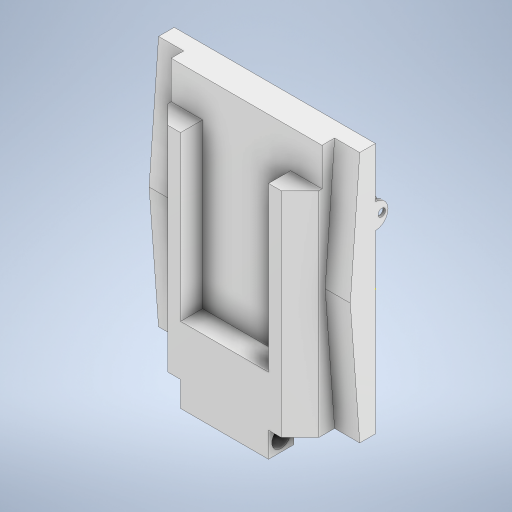
# Autodesk Inventor part: Hebeteil
Saved by Autodesk Inventor 2023 (Build 270158000, 158)
## iProperties
Created: 2024-02-03
Part Number: Hebeteil
Material: Acetalharz, Weiß
Document SubType Name: Modeling
Designer: jefar
Density: 1.425 g/cm^3
Appearance: Glatt - Weiß
Mass: 1.50722e+08 g
Surface Area: 2.46257e+06 cm^2
Volume: 1.0577e+08 cm^3
Author: jefar
Autodesk Inventor part; units mm, degrees
ref_plane "YZ Plane" through (0, 0, 0) normal (1, 0, 0) x (0, 1, 0)
sketch "Skizze1" plane through (0, 0, 0) normal (0, 0, 1) x (1, 0, 0)
  line L0 (-5600, 0) -> (5600, 0) construction
  line L1 (0, -7000) -> (0, 7000) construction
  line L2 (-4000, -5000) -> (4000, -5000)
  line L3 (4000, -5000) -> (4000, 5000)
  line L4 (4000, 5000) -> (-4000, 5000)
  line L5 (-4000, 5000) -> (-4000, -5000)
  line L6 (-4000, -5000) -> (4000, 5000) construction
  line L7 (4000, -5000) -> (-4000, 5000) construction
  point P0 (0, 0)
  dimension "d0" = 8000
  dimension "d1" = 10000
  constraints: 12 end point, 2 midpoint, 2 parallel, 1 horizontal, 1 perpendicular
  measures "d0" distance of L4.end L3.end
  measures "d1" distance of L3.end L2.end
extrude "Extrusion1" add sketch "Skizze1" along normal blind 2000
sketch "Skizze2" plane through (-4000, 5000, 0) normal (0, 1, 0) x (1, 0, 0)
  line L0 (0, 0) -> (0, -1250)
  line L1 (0, -1250) -> (0, 0)
  line L2 (0, -1250) -> (1000, -1250)
  line L3 (8000, 0) -> (8000, -2000) construction
  line L4 (0, 0) -> (0, -2000) projected
  line L5 (1000, -1250) -> (1000, -2000)
  line L6 (8000, -2000) -> (0, -2000) construction
  line L7 (1000, -2000) -> (4000, -2000)
  line L8 (8000, 0) -> (8000, -1250)
  line L9 (8000, -1250) -> (7000, -1250)
  line L10 (7000, -1250) -> (7000, -2000)
  line L11 (8000, 0) -> (0, 0) projected
  line L12 (8000, 0) -> (0, 0)
  line L13 (7000, -2000) -> (4000, -2000)
  line L14 (0, -1250) -> (0, -2000)
  line L15 (0, -2000) -> (1000, -2000)
  line L16 (8000, -1250) -> (8000, -2000)
  line L17 (7000, -2000) -> (8000, -2000)
  line L18 (8000, -2000) -> (8000, -1250)
  point P0 (4000, 0)
  dimension "d4" = 750
  dimension "d5" = 1250
  dimension "d7" = 1000
  constraints: 30 end point, 5 collinear, 2 horizontal, 1 midpoint, 1 point on line, 1 vertical
  measures "d4" distance of L0.end L4.end
  measures "d5" distance of L0.end L0.start
  measures "d7" distance of L0.end L2.end
extrude "Extrusion2" cut sketch "Skizze2" against normal through all contours L2 L5 L15 L4 | L16 L17 L10 L9
chamfer "Fase1" distance 750 angle 45 2 edges at (-3000, 0, 2000) (3000, 0, 2000)
sketch "Skizze3" plane through (4000, -5000, 0) normal (1, 0, 0) x (0, 0, -1)
  line L0 (0, 10000) -> (0, 8000)
  arc A0 (0, 7000) -> (0, 8000) centre (0, 7500) ccw
  line L1 (0, 7000) -> (0, 0)
  line L2 (0, 8000) -> (0, 7000)
  line L3 (0, 0) -> (0, 10000) projected
  point P0 (0, 5000)
  dimension "d16" = 2000
  dimension "d17" = 7000
  constraints: 6 end point, 2 collinear, 2 point on circle, 2 point on line, 1 centre point
  measures "d16" distance of L0.start L0.end
  measures "d17" distance of L1.start L1.end
extrude "Extrusion3" add sketch "Skizze3" against normal blind 500
sketch "Skizze4" plane through (0, 0, 0) normal (0, 0, -1) x (-1, 0, 0)
  point P0 (0, 0)
sketch "Skizze5" plane through (-4000, -5000, 0) normal (-1, 0, 0) x (0, 0, 1)
  line L0 (0, 8000) -> (0, 7000) projected
  arc A0 (0, 8000) -> (0, 7000) centre (0, 7500) ccw
  line L1 (0, 7000) -> (0, 8000)
  point P0 (0, 5000)
  constraints: 2 end point, 2 point on circle, 1 centre point, 1 midpoint
extrude "Extrusion4" add sketch "Skizze5" against normal blind 500
ref_plane "Arbeitsebene1" through (4000, 2000, 0) normal (0, 1, 0) x (1, 0, 0)
sketch "Skizze6" plane through (4000, 2000, 0) normal (0, 1, 0) x (1, 0, 0)
  line L0 (-100, 0) -> (-400, 0)
  line L1 (0, 0) -> (0, -1250) projected
  line L2 (-7900, 0) -> (-7600, 0)
  line L3 (0, 500) -> (-500, 500) projected
  line L4 (-100, 0) -> (-400, 0)
  line L5 (-400, 0) -> (-400, 500)
  line L6 (-400, 500) -> (-100, 500)
  line L7 (-100, 500) -> (-100, 0)
  line L8 (-8000, 500) -> (-7500, 500) construction
  line L9 (-7600, 0) -> (-7900, 0)
  line L10 (-7900, 0) -> (-7900, 500)
  line L11 (-7900, 500) -> (-7600, 500)
  line L12 (-7600, 500) -> (-7600, 0)
  point P0 (-4000, 0)
  point P1 (-8000, 0)
  dimension "d22" = 300
  dimension "d23" = 100
  dimension "d25" = 300
  constraints: 20 end point, 4 parallel, 2 horizontal, 2 perpendicular, 2 point on line
  measures "d22" distance of L0.start L0.end
  measures "d23" distance from line of L1 L0.start
  measures "d25" distance of L2.start L2.end
extrude "Extrusion5" cut sketch "Skizze6" along normal through all
sketch "Skizze7" plane through (0, 0, 2000) normal (0, 0, 1) x (1, 0, 0)
  line L0 (-2250, -5000) -> (2250, -5000) construction
  line L1 (-1750, 5000) -> (1750, 5000)
  line L2 (1750, 5000) -> (1750, -5000)
  line L3 (1750, -5000) -> (-1750, -5000)
  line L4 (-1750, -5000) -> (-1750, 5000)
  line L5 (-1750, 5000) -> (1750, -5000) construction
  line L6 (1750, 5000) -> (-1750, -5000) construction
  point P0 (0, 0)
  dimension "d28" = 3500
  constraints: 12 end point, 2 midpoint, 2 parallel, 1 horizontal, 1 perpendicular, 1 point on line
  measures "d28" distance of L2.end L3.end
extrude "Extrusion6" cut sketch "Skizze7" against normal blind 1000
sketch "Skizze8" plane through (-4000, -5000, 1250) normal (-1, 0, 0) x (0, 0, 1)
  line L0 (-1250, 0) -> (0, 0) projected
  line L1 (-625, 0) -> (-250, 5000)
  line L2 (-250, 10000) -> (-250, 0) projected
  line L3 (-250, 5000) -> (-625, 10000)
  line L4 (-1250, 10000) -> (0, 10000) projected
  line L5 (-1250, 7000) -> (-1250, 0) construction
  line L6 (0, 10000) -> (0, 0) projected
  line L7 (-1250, 0) -> (0, 0)
  line L8 (750, 10000) -> (0, 10000) construction
  line L9 (0, 0) -> (0, 10000)
  line L10 (0, 10000) -> (-1250, 10000)
  line L11 (-250, 0) -> (-250, 10000)
  point P0 (-1250, 5000)
  constraints: 12 end point, 3 midpoint, 2 perpendicular, 1 collinear, 1 horizontal
extrude "Extrusion7" cut sketch "Skizze8" against normal blind 1000 contours L1 L2 L0 | L3 L4 L2
sketch "Skizze9" plane through (-4000, -5000, 1250) normal (-1, 0, 0) x (0, 0, 1)
  line L0 (0, 0) -> (0, 10000) projected
  line L1 (-250, 0) -> (0, 0)
  line L2 (0, 0) -> (0, 10000)
  line L3 (0, 10000) -> (-250, 10000)
  line L4 (-250, 10000) -> (-250, 0)
  point P0 (-1250, 5000)
  constraints: 8 end point, 2 parallel, 1 horizontal, 1 perpendicular
extrude "Extrusion8" cut sketch "Skizze9" against normal blind 1000
sketch "Skizze10" plane through (4000, -5000, 1250) normal (1, 0, 0) x (0, 0, -1)
  line L0 (250, 5000) -> (625, 10000) projected
  line L1 (625, 0) -> (250, 5000) projected
  line L2 (625, 10000) -> (250, 5000)
  line L3 (250, 5000) -> (625, 0)
  line L4 (1250, 0) -> (0, 0) construction
  line L5 (625, 10000) -> (1250, 10000)
  line L6 (1250, 10000) -> (0, 10000) projected
  line L7 (625, 10000) -> (0, 10000)
  line L8 (0, 10000) -> (0, 0) projected
  line L9 (0, 10000) -> (0, 0)
  line L10 (0, 0) -> (625, 0)
  point P0 (1250, 5000)
  constraints: 12 end point, 1 collinear, 1 horizontal, 1 midpoint, 1 perpendicular
extrude "Extrusion9" cut sketch "Skizze10" against normal blind 1000
sketch "Skizze11" plane through (-4000, -5000, 0) normal (-1, 0, 0) x (0, 0, 1)
  circle A0 centre (-250, 7500) radius 150
  point P0 (0, 5000)
  dimension "d37" = 300
  constraints: 1 centre point
  measures "d37" diameter of A0
extrude "Extrusion10" cut sketch "Skizze11" against normal through all
sketch "Skizze12" plane through (-4000, -5000, 0) normal (0, -1, 0) x (1, 0, 0)
  line L0 (5750, 1000) -> (5750, 2000) projected
  line L1 (5750, 1000) -> (2250, 1000) projected
  line L2 (5750, 2000) -> (2250, 2000)
  line L3 (2250, 2000) -> (2250, 1000)
  line L4 (2250, 1000) -> (5750, 1000)
  line L5 (5750, 1000) -> (5750, 2000)
  point P0 (4000, 0)
  constraints: 8 end point, 2 parallel, 1 horizontal, 1 perpendicular
extrude "Extrusion11" add sketch "Skizze12" along normal blind 1000
sketch "Skizze13" plane through (-4000, 5000, 0) normal (0, 1, 0) x (1, 0, 0)
  line L0 (5750, -2000) -> (2250, -2000) projected
  line L1 (2250, -1000) -> (5750, -1000) projected
  line L2 (2250, -2000) -> (5750, -2000)
  line L3 (5750, -2000) -> (5750, -1000)
  line L4 (5750, -1000) -> (2250, -1000)
  line L5 (2250, -1000) -> (2250, -2000)
  point P0 (4000, 0)
  constraints: 8 end point, 2 parallel, 1 horizontal, 1 perpendicular
extrude "Extrusion12" add sketch "Skizze13" against normal blind 10000
sketch "Skizze14" plane through (1750, -5000, 2000) normal (1, 0, 0) x (0, 0, -1)
  line L0 (1000, -1000) -> (0, -1000) construction
  line L1 (0, 0) -> (0, -1000) construction
  circle A0 centre (500, -500) radius 375
  point P0 (2000, 5000)
  dimension "d44" = 750
  constraints: 1 centre point
  measures "d44" diameter of A0
extrude "Extrusion13" cut sketch "Skizze14" against normal blind 10000
sketch "Skizze15" plane through (4000, -5000, 0) normal (1, 0, 0) x (0, 0, -1)
  point P0 (0, 5000)
sketch "Skizze16" plane through (4000, -5000, 0) normal (1, 0, 0) x (0, 0, -1)
  point P0 (0, 5000)
sketch "Skizze17" plane through (-4000, 5000, 0) normal (0, 1, 0) x (1, 0, 0)
  line L0 (5750, -1125) -> (2250, -1125) projected
  line L1 (5750, -1000) -> (5750, -2000) projected
  line L2 (2250, -1125) -> (5750, -1125)
  line L3 (5750, -1125) -> (5750, -2000)
  line L4 (5750, -2000) -> (2250, -2000)
  line L5 (2250, -2000) -> (2250, -1125)
  point P0 (4000, 0)
  constraints: 8 end point, 2 parallel, 1 horizontal, 1 perpendicular, 1 point on line
extrude "Extrusion14" cut sketch "Skizze17" against normal blind 8000
ref_plane "Arbeitsebene2" through (2000, 5000, 2000) normal (0, 0, 1) x (1, 0, 0)
sketch "Skizze18" plane through (-1750, 5000, 1125) normal (0, 0, 1) x (1, 0, 0)
  line L0 (4750, 0) -> (4750, -10000) projected
  line L1 (-1250, 0) -> (4750, 0)
  line L2 (4750, 0) -> (4750, -1500)
  line L3 (4750, -1500) -> (-1250, -1500)
  line L4 (-1250, -1500) -> (-1250, 0)
  line L5 (-500, 0) -> (-1250, 0) projected
  line L6 (-1250, 0) -> (4750, 0)
  line L7 (4750, 0) -> (4750, -1500)
  line L8 (4750, -1500) -> (-1250, -1500)
  line L9 (-1250, -1500) -> (-1250, 0)
  point P0 (1750, -5000)
  dimension "d49" = 1500
  constraints: 16 end point, 4 parallel, 2 horizontal, 2 perpendicular, 1 point on line
  measures "d49" distance of L1.end L2.end
extrude "Extrusion15" cut sketch "Skizze18" along normal blind 2000
